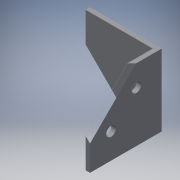
# Autodesk Inventor part: rail gusset
Saved by Autodesk Inventor 2016 (Build 200138000, 138)
## iProperties
Created: 2016-02-08
Part Number: rail gusset
Material: Aluminum 6061
Document SubType Name: Modeling
Designer: gus
Density: 2.7 g/cm^3
Appearance: Aluminum - Flat
Author: gus
Autodesk Inventor part; units mm, degrees
ref_plane "YZ Plane" through (0, 0, 0) normal (1, 0, 0) x (0, 1, 0)
ref_plane "XZ Plane" through (0, 0, 0) normal (0, 1, 0) x (-1, 0, 0)
ref_plane "XY Plane" through (0, 0, 0) normal (0, 0, 1) x (1, 0, 0)
sketch "Sketch1" plane through (0, 0, 0) normal (0, 1, 0) x (-1, 0, 0)
  line L0 (0, 0) -> (0, 50.8)
  line L1 (0, 50.8) -> (3.175, 50.8)
  line L2 (3.175, 50.8) -> (3.175, 3.175)
  line L3 (3.175, 3.175) -> (50.8, 3.175)
  line L4 (50.8, 3.175) -> (50.8, 0)
  line L5 (50.8, 0) -> (0, 0)
  dimension "d0" = 50.8
  dimension "d1" = 3.175
  dimension "d2" = 47.625
  dimension "d3" = 47.625
  constraints: 12 end point, 5 perpendicular, 1 vertical
  measures "d0" distance of L0.start L0.end
  measures "d1" distance of L0.end L1.end
  measures "d2" distance of L1.end L2.end
  measures "d3" distance of L2.end L3.end
extrude "Extrusion1" add sketch "Sketch1" along normal blind 50.8
sketch "Sketch2" plane through (-3.175, 0, 3.175) normal (-1, 0, 0) x (0, 0, 1)
  line L0 (17.867, 50.8) -> (47.625, 21.042)
  line L1 (0, 50.8) -> (47.625, 50.8) projected
  line L2 (47.625, 0) -> (47.625, 50.8) projected
  line L3 (47.625, 0) -> (47.625, 50.8) projected
  line L4 (47.625, 21.042) -> (47.625, 50.8)
  line L5 (47.625, 50.8) -> (-3.175, 50.8) projected
  line L6 (47.625, 50.8) -> (17.867, 50.8)
  line L7 (-3.175, 0) -> (47.625, 0) projected
  line L8 (-3.175, 0) -> (-3.175, 50.8) projected
  dimension "d6" = 50.8
  dimension "d7" = 45
  constraints: 6 end point, 3 point on line, 2 collinear
  measures "d6" distance from line of L7.start L0
  measures "d7" angle of L1 L0
extrude "Extrusion3" cut sketch "Sketch2" against normal blind 3.175 contours L1 L2 L0
sketch "Sketch3" plane through (-3.175, 0, 3.175) normal (-1, 0, 0) x (0, 0, 1)
  circle A0 centre (14.7855, 35.921) radius 3.3734
  circle A1 centre (32.746, 17.9605) radius 3.3734
  line L0 (47.625, 21.042) -> (17.867, 50.8) projected
  line L1 (14.7855, 35.921) -> (-0.0935, 50.8) construction
  line L2 (0, 50.8) -> (17.867, 50.8) projected
  line L3 (32.746, 17.9605) -> (47.625, 3.0815) construction
  line L4 (47.625, -14.879) -> (47.625, 21.042) construction
  line L5 (47.625, 0) -> (47.625, 21.042) construction
  point P0 (-3.175, 0)
  dimension "d18" = 6.7469
  dimension "d19" = 6.7469
  dimension "d20" = 12.7
  dimension "d21" = 12.7
  dimension "d22" = 25.4
  dimension "d23" = 21.042
  constraints: 6 end point, 2 centre point, 2 parallel, 2 point on line, 1 collinear, 1 midpoint
  measures "d18" diameter of A0
  measures "d19" diameter of A1
  measures "d20" distance from line of L0 L1.start
  measures "d21" distance from line of L0 L3.start
  measures "d22" distance of L1.start L3.start
  measures "d23" distance of L3.start L3.end
extrude "Extrusion4" cut sketch "Sketch3" against normal blind 3.175
sketch "Sketch4" plane through (0, 0, 0) normal (0, 0, -1) x (-1, 0, 0)
  circle A0 centre (12.7, 38.1) radius 3.3734
  circle A1 centre (38.1, 38.1) radius 3.3734
  line L0 (50.8, 0) -> (50.8, 50.8) projected
  line L1 (0, 50.8) -> (50.8, 50.8) projected
  point P0 (0, 0)
  dimension "d26" = 6.7469
  dimension "d27" = 12.7
  dimension "d28" = 12.7
  dimension "d29" = 12.7
  dimension "d30" = 38.1
  constraints: 2 centre point, 1 equal radius
  measures "d26" diameter of A1
  measures "d27" distance from line of L0 A1.centre
  measures "d28" distance from line of L1 A1.centre
  measures "d29" distance from line of L1 A0.centre
  measures "d30" distance from line of L0 A0.centre
extrude "Extrusion5" cut sketch "Sketch4" against normal blind 3.175
body "Solid1"
